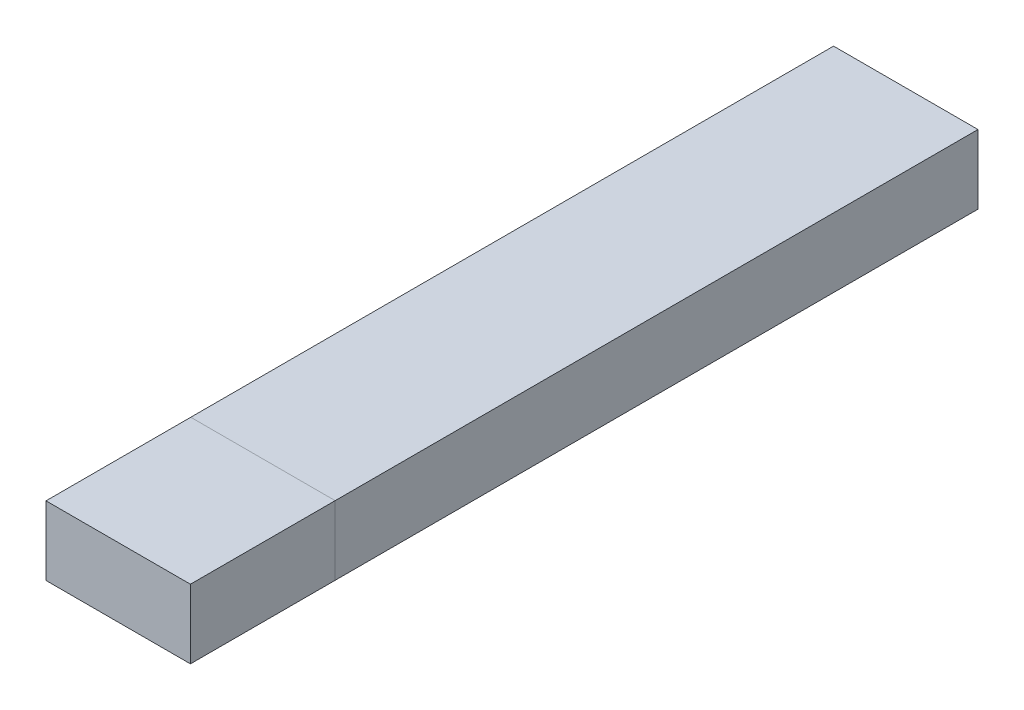
# Autodesk Inventor part: Contenedor3
Saved by Autodesk Inventor 2020.3 (Build 243373000, 373)
## iProperties
Created: 2020-09-22
Part Number: Contenedor3
Material: ABS Plastic
Document SubType Name: Modeling
Designer: juanp
Density: 1.06 g/cm^3
Appearance: Smooth - White
Mass: 443.385 g
Surface Area: 3011.82 cm^2
Volume: 418.287 cm^3
Author: juanp
Autodesk Inventor part; units mm, degrees
sketch "Sketch1" plane through (0, 0, 0) normal (0, 1, 0) x (-1, 0, 0)
  line L0 (0, 0) -> (0, -358.09) construction
  line L1 (42, 13.6996) -> (0, 13.6996)
  line L2 (0, 13.6996) -> (0, -13.6996)
  line L3 (0, -13.6996) -> (42, -13.6996)
  line L4 (42, -13.6996) -> (42, 13.6996)
  line L5 (42, -15.6996) -> (0, -15.6996)
  line L6 (0, -15.6996) -> (0, -43.0987)
  line L7 (0, -43.0987) -> (42, -43.0987)
  line L8 (42, -43.0987) -> (42, -15.6996)
  line L9 (42, -45.0987) -> (0, -45.0987)
  line L10 (0, -45.0987) -> (0, -72.4978)
  line L11 (0, -72.4978) -> (42, -72.4978)
  line L12 (42, -72.4978) -> (42, -45.0987)
  line L13 (42, -105.897) -> (0, -105.897)
  line L14 (0, -105.897) -> (0, -133.2961)
  line L15 (0, -133.2961) -> (42, -133.2961)
  line L16 (42, -133.2961) -> (42, -105.897)
  line L17 (42, -135.2961) -> (0, -135.2961)
  line L18 (0, -135.2961) -> (0, -162.6952)
  line L19 (0, -162.6952) -> (42, -162.6952)
  line L20 (42, -162.6952) -> (42, -135.2961)
  line L21 (42, -76.4978) -> (0, -76.4978)
  line L22 (0, -76.4978) -> (0, -103.897)
  line L23 (0, -103.897) -> (42, -103.897)
  line L24 (42, -103.897) -> (42, -76.4978)
  line L25 (21, -13.6996) -> (21, -15.6996)
  line L26 (21, -43.0987) -> (21, -45.0987)
  line L27 (21, -103.897) -> (21, -105.897)
  line L28 (21, -133.2961) -> (21, -135.2961)
  line L29 (42, -166.6952) -> (0, -166.6952)
  line L30 (0, -166.6952) -> (0, -194.0943)
  line L31 (0, -194.0943) -> (42, -194.0943)
  line L32 (42, -194.0943) -> (42, -166.6952)
  line L33 (42, -196.0943) -> (0, -196.0943)
  line L34 (0, -196.0943) -> (0, -223.4935)
  line L35 (0, -223.4935) -> (42, -223.4935)
  line L36 (42, -223.4935) -> (42, -196.0943)
  line L37 (42, -225.4935) -> (0, -225.4935)
  line L38 (0, -225.4935) -> (0, -252.8926)
  line L39 (0, -252.8926) -> (42, -252.8926)
  line L40 (42, -252.8926) -> (42, -225.4935)
  line L41 (42, -286.2917) -> (0, -286.2917)
  line L42 (0, -286.2917) -> (0, -313.6909)
  line L43 (0, -313.6909) -> (42, -313.6909)
  line L44 (42, -313.6909) -> (42, -286.2917)
  line L45 (42, -315.6909) -> (0, -315.6909)
  line L46 (0, -315.6909) -> (0, -343.09)
  line L47 (0, -343.09) -> (42, -343.09)
  line L48 (42, -343.09) -> (42, -315.6909)
  line L49 (42, -256.8926) -> (0, -256.8926)
  line L50 (0, -256.8926) -> (0, -284.2917)
  line L51 (0, -284.2917) -> (42, -284.2917)
  line L52 (42, -284.2917) -> (42, -256.8926)
  line L53 (21, -194.0943) -> (21, -196.0943)
  line L54 (21, -223.4935) -> (21, -225.4935)
  line L55 (21, -284.2917) -> (21, -286.2917)
  line L56 (21, -313.6909) -> (21, -315.6909)
  line L57 (88, 15.6996) -> (-2, 15.6996)
  line L58 (-2, 15.6996) -> (-2, -475.09)
  line L59 (-2, -475.09) -> (88, -475.09)
  line L60 (88, -475.09) -> (88, 15.6996)
  line L61 (44, 0) -> (44, -362.09) construction
  line L62 (86, 13.6996) -> (44, 13.6996)
  line L63 (44, 13.6996) -> (44, -13.6996)
  line L64 (44, -13.6996) -> (86, -13.6996)
  line L65 (86, -13.6996) -> (86, 13.6996)
  line L66 (86, -15.6996) -> (44, -15.6996)
  line L67 (44, -15.6996) -> (44, -43.0987)
  line L68 (44, -43.0987) -> (86, -43.0987)
  line L69 (86, -43.0987) -> (86, -15.6996)
  line L70 (86, -45.0987) -> (44, -45.0987)
  line L71 (44, -45.0987) -> (44, -72.4978)
  line L72 (44, -72.4978) -> (86, -72.4978)
  line L73 (86, -72.4978) -> (86, -45.0987)
  line L74 (86, -105.897) -> (44, -105.897)
  line L75 (44, -105.897) -> (44, -133.2961)
  line L76 (44, -133.2961) -> (86, -133.2961)
  line L77 (86, -133.2961) -> (86, -105.897)
  line L78 (86, -135.2961) -> (44, -135.2961)
  line L79 (44, -135.2961) -> (44, -162.6952)
  line L80 (44, -162.6952) -> (86, -162.6952)
  line L81 (86, -162.6952) -> (86, -135.2961)
  line L82 (86, -76.4978) -> (44, -76.4978)
  line L83 (44, -76.4978) -> (44, -103.897)
  line L84 (44, -103.897) -> (86, -103.897)
  line L85 (86, -103.897) -> (86, -76.4978)
  line L86 (65, -13.6996) -> (65, -15.6996)
  line L87 (65, -43.0987) -> (65, -45.0987)
  line L88 (65, -103.897) -> (65, -105.897)
  line L89 (65, -133.2961) -> (65, -135.2961)
  line L90 (44, -225.4935) -> (44, -252.8926)
  line L91 (86, -252.8926) -> (86, -225.4935)
  line L92 (86, -256.8926) -> (44, -256.8926)
  line L93 (44, -256.8926) -> (44, -284.2917)
  line L94 (86, -284.2917) -> (86, -256.8926)
  line L95 (44, -252.8926) -> (86, -252.8926)
  line L96 (86, -166.6952) -> (44, -166.6952)
  line L97 (44, -166.6952) -> (44, -194.0943)
  line L98 (44, -194.0943) -> (86, -194.0943)
  line L99 (86, -194.0943) -> (86, -166.6952)
  line L100 (86, -225.4935) -> (44, -225.4935)
  line L101 (65, -223.4935) -> (65, -225.4935)
  line L102 (44, -223.4935) -> (86, -223.4935)
  line L103 (86, -223.4935) -> (86, -196.0943)
  line L104 (86, -196.0943) -> (44, -196.0943)
  line L105 (44, -196.0943) -> (44, -223.4935)
  line L106 (65, -194.0943) -> (65, -196.0943)
  line L107 (86, -286.2917) -> (44, -286.2917)
  line L108 (44, -286.2917) -> (44, -313.6909)
  line L109 (44, -313.6909) -> (86, -313.6909)
  line L110 (86, -313.6909) -> (86, -286.2917)
  line L111 (44, -284.2917) -> (86, -284.2917)
  line L112 (65, -313.6909) -> (65, -315.6909)
  line L113 (86, -315.6909) -> (44, -315.6909)
  line L114 (86, -343.09) -> (86, -315.6909)
  line L115 (44, -343.09) -> (86, -343.09)
  line L116 (44, -315.6909) -> (44, -343.09)
  line L117 (65, -284.2917) -> (65, -286.2917)
  line L118 (65, 13.6996) -> (65, 15.6996)
  line L119 (65, -72.4978) -> (65, -76.4978)
  line L120 (21, -72.4978) -> (21, -76.4978)
  line L121 (65, -162.6952) -> (65, -166.6952)
  line L122 (21, -162.6952) -> (21, -166.6952)
  line L123 (65, -252.8926) -> (65, -256.8926)
  line L124 (21, -252.8926) -> (21, -256.8926)
  line L125 (0, -347.09) -> (86, -347.09)
  line L126 (86, -347.09) -> (86, -377.09)
  line L127 (86, -377.09) -> (0, -377.09)
  line L128 (0, -377.09) -> (0, -347.09)
  line L129 (86, -362.09) -> (0, -362.09) construction
  line L130 (65, -343.09) -> (65, -347.09)
  line L131 (21, -343.09) -> (21, -347.09)
  line L132 (0, -379.09) -> (86, -379.09)
  line L133 (86, -379.09) -> (86, -409.09)
  line L134 (86, -409.09) -> (0, -409.09)
  line L135 (0, -409.09) -> (0, -379.09)
  line L136 (0, -411.09) -> (86, -411.09)
  line L137 (86, -411.09) -> (86, -441.09)
  line L138 (86, -441.09) -> (0, -441.09)
  line L139 (0, -441.09) -> (0, -411.09)
  line L140 (43, -377.09) -> (43, -379.09)
  line L141 (43, -409.09) -> (43, -411.09)
  line L142 (0, -443.09) -> (86, -443.09)
  line L143 (86, -443.09) -> (86, -473.09)
  line L144 (86, -473.09) -> (0, -473.09)
  line L145 (0, -473.09) -> (0, -443.09)
  line L146 (43, -441.09) -> (43, -443.09)
  line L147 (43, -475.09) -> (43, -473.09)
  point P0 (0, -29.3991)
  point P1 (0, -58.7983)
  point P2 (0, -119.5965)
  point P3 (0, -148.9957)
  point P4 (0, -90.1974)
  point P5 (0, -180.3948)
  point P6 (0, -209.7939)
  point P7 (0, -239.193)
  point P8 (0, -299.9913)
  point P9 (0, -329.3904)
  point P10 (0, -270.5922)
  point P11 (44, -29.3991)
  point P12 (44, -58.7983)
  point P13 (44, -119.5965)
  point P14 (44, -148.9957)
  point P15 (44, -90.1974)
  point P16 (44, -239.193)
  point P17 (44, -270.5922)
  point P18 (44, -180.3948)
  point P19 (44, -209.7939)
  point P20 (44, -299.9913)
  point P21 (44, -329.3904)
  point P22 (65, -254.8926)
  point P23 (0, -458.09)
  dimension "d7" = 2
  dimension "d8" = 2
  dimension "d12" = 2
  dimension "d13" = 2
  dimension "d14" = 90
  dimension "d15" = 2
  dimension "d16" = 4
  dimension "d17" = 4
  dimension "d18" = 4
  dimension "d25" = 30
  dimension "d27" = 27.3991
  dimension "d28" = 92.1974
  dimension "d30" = 458.09
  constraints: 292 end point, 83 midpoint, 73 equal length, 58 parallel, 32 perpendicular, 29 horizontal, 6 point on line, 5 collinear, 1 coincident, 29 other
  measures "d7" distance between parallel lines of L58 L2
  measures "d8" distance between parallel lines of L57 L1
  measures "d12" distance of L118.start L118.end
  measures "d13" distance between parallel lines of L60 L73
  measures "d14" distance of L58.end L59.end
  measures "d15" distance between parallel lines of L4 L63
  measures "d16" distance of L120.start L120.end
  measures "d17" distance of L122.start L122.end
  measures "d18" distance of L124.start L124.end
  measures "d25" distance of L125.end L126.end
  measures "d27" distance of L48.start L45.start
  measures "d28" distance from line of point (65, -254.893) L125
  measures "d30" distance of point (0, 0) point (0, -458.09)
extrude "Extrusion1" add sketch "Sketch1" along normal blind 40 contours L60 L59 L147 L144 L143 L142 L146 L138 L137 L136 L141 L134 L133 L132 L140 L127 L126 L125 L130 L115 L114 L113 L112 L109 L110 L107 L117 L111 L94 L92 L123 L95 L91 L100 L101 L102 L103 L104 L106 L98 L99 L96 L121 L80 L81 L78 L89 L76 L77 L74 L88 L84 L85 L82 L119 L72 L73 L70 L87 L68 L69 L66 L86 L64 L65 L62 L118 L57 | L118 L62 L63 L64 L86 L66 L67 L68 L87 L70 L71 L72 L119 L82 L83 L84 L88 L74 L75 L76 L89 L78 L79 L80 L121 L96 L97 L98 L106 L104 L105 L102 L101 L100 L90 L95 L123 L92 L93 L111 L117 L107 L108 L109 L112 L113 L116 L115 L130 L125 L128 L127 L140 L132 L135 L134 L141 L136 L139 L138 L146 L142 L145 L144 L147 L59 L58 L57
sketch "Sketch2" plane through (0, 40, 0) normal (0, 1, 0) x (1, 0, 0)
  line L0 (2, -15.6996) -> (2, 475.09) projected
  line L1 (-88, -15.6996) -> (2, -15.6996) projected
  line L2 (-88, 475.09) -> (-88, -15.6996) projected
  line L3 (2, 475.09) -> (-88, 475.09) projected
  point P0 (0, 0)
extrude "Extrusion2" add sketch "Sketch2" along normal blind 3
fillet "Fillet1" radius 5 192 edges at (-42, 20, -45.0987) (0, 20, -45.0987) (-42, 20, -43.0987) (0, 20, -15.6996) (-21, 40, 13.6996) (-44, 20, -103.897) (-44, 20, -105.897) (-44, 20, -133.2961) (-86, 20, -133.2961) (-86, 20, -105.897) (-86, 20, -76.4978) (0, 20, -72.4978) (-21, 40, -43.0987) (-86, 20, -13.6996) (-86, 20, -15.6996) (-44, 20, -15.6996) (-86, 20, 13.6996) (-44, 20, -13.6996) (-44, 20, 13.6996) (-42, 20, -15.6996) (-86, 40, -270.5922) (-42, 40, -299.9913) (-65, 40, -286.2917) (-86, 40, -299.9913) (-44, 40, -299.9913) (-42, 40, -270.5922) (-44, 40, -270.5922) (-42, 40, -239.193) (-65, 40, -284.2917) (-65, 40, -313.6909) (0, 20, -43.0987) (-42, 40, -29.3991) (-21, 40, -15.6996) (-42, 20, -13.6996) (0, 20, -13.6996) (0, 20, 13.6996) (0, 20, -162.6952) (0, 20, -135.2961) (0, 20, -133.2961) (-42, 20, -162.6952) (-42, 20, -135.2961) (-86, 20, -135.2961) (-44, 20, -135.2961) (-86, 20, -162.6952) (-44, 20, -162.6952) (-86, 20, -166.6952) (-44, 40, -180.3948) (0, 20, -194.0943) (-42, 20, -166.6952) (-42, 20, -194.0943) (0, 20, -166.6952) (-44, 20, -43.0987) (-44, 20, -45.0987) (-44, 20, -72.4978) (-44, 20, -76.4978) (-86, 20, -43.0987) (-86, 20, -45.0987) (-21, 40, -13.6996) (-86, 20, -72.4978) (-42, 20, 13.6996) (-86, 20, -103.897) (-65, 40, -223.4935) (-86, 40, -209.7939) (-65, 40, -196.0943) (-44, 40, -209.7939) (-65, 40, -166.6952) (-65, 40, -194.0943) (-86, 40, -180.3948) (-65, 40, -162.6952) (-44, 20, -166.6952) (-86, 20, -194.0943) (-86, 20, -196.0943) (-86, 20, -223.4935) (-44, 20, -223.4935) (-44, 20, -194.0943) (0, 20, -223.4935) (0, 20, -196.0943) (-42, 20, -196.0943) (-42, 20, -223.4935) (-42, 40, -180.3948) (0, 40, -180.3948) (-21, 40, -196.0943) (-21, 40, -223.4935) (-42, 40, -209.7939) (0, 40, -209.7939) (-21, 40, -225.4935) (0, 40, -239.193) (-21, 40, -194.0943) (-44, 20, -196.0943) (-86, 20, -225.4935) (-44, 20, -225.4935) (-86, 20, -252.8926) (-44, 20, -252.8926) (-86, 20, -256.8926) (-65, 40, -256.8926) (-65, 40, -252.8926) (-86, 40, -239.193) (-44, 40, -239.193) (-65, 40, -225.4935) (0, 20, -252.8926) (0, 20, -225.4935) (-42, 20, -252.8926) (-42, 20, -225.4935) (-86, 20, -284.2917) (0, 20, -313.6909) (0, 20, -286.2917) (-42, 20, -286.2917) (-42, 20, -313.6909) (-44, 20, -256.8926) (-44, 20, -284.2917) (-44, 20, -286.2917) (-44, 20, -313.6909) (-86, 20, -313.6909) (-86, 20, -286.2917) (-42, 20, -315.6909) (-42, 20, -343.09) (0, 20, -315.6909) (-44, 20, -315.6909) (-86, 20, -315.6909) (-44, 20, -343.09) (-86, 20, -343.09) (0, 20, -343.09) (-21, 40, -252.8926) (-21, 40, -256.8926) (0, 40, -270.5922) (-21, 40, -284.2917) (0, 40, -299.9913) (-21, 40, -286.2917) (-21, 40, -313.6909) (-21, 40, -315.6909) (-65, 40, -315.6909) (-42, 40, -329.3904) (-21, 40, -343.09) (0, 40, -329.3904) (-44, 40, -329.3904) (-86, 40, -329.3904) (-65, 40, -343.09) (0, 20, -284.2917) (0, 20, -256.8926) (-42, 20, -256.8926) (-42, 20, -284.2917) (-65, 40, -72.4978) (-86, 40, -58.7983) (-65, 40, -45.0987) (-44, 40, -58.7983) (-65, 40, -43.0987) (-86, 40, -29.3991) (-65, 40, -15.6996) (-44, 40, -29.3991) (-65, 40, -13.6996) (-86, 40, 0) (-65, 40, 13.6996) (-44, 40, 0) (-44, 40, -148.9957) (-86, 40, -148.9957) (-65, 40, -133.2961) (-65, 40, -135.2961) (-86, 40, -119.5965) (-44, 40, -119.5965) (-65, 40, -105.897) (-21, 40, -133.2961) (-21, 40, -135.2961) (0, 40, -148.9957) (-21, 40, -162.6952) (-42, 40, -148.9957) (-21, 40, -105.897) (0, 40, -119.5965) (-42, 40, -119.5965) (-21, 40, -103.897) (-21, 40, -76.4978) (-42, 40, -90.1974) (0, 40, -90.1974) (-21, 40, -166.6952) (-42, 20, -72.4978) (-42, 20, -133.2961) (0, 20, -105.897) (-42, 20, -105.897) (0, 20, -103.897) (-42, 20, -103.897) (-21, 40, -45.0987) (0, 40, -58.7983) (-42, 40, -58.7983) (-21, 40, -72.4978) (0, 40, -29.3991) (-42, 40, 0) (0, 40, 0) (0, 20, -76.4978) (-42, 20, -76.4978) (-86, 40, -90.1974) (-65, 40, -76.4978) (-44, 40, -90.1974) (-65, 40, -103.897)
ref_plane "Work Plane1" through (-88, 0, -229.6952) normal (0, 0, 1) x (1, 0, 0)
ref_plane "Work Plane2" through (-43, 0, 15.6996) normal (1, 0, 0) x (0, 0, -1)
ref_plane "Work Plane3" through (-43, 0, 15.6996) normal (1, 0, 0) x (0, 0, -1)
ref_plane "Work Plane4" through (-81, 0, -74.4978) normal (0, 0, 1) x (1, 0, 0)
ref_plane "Work Plane5" through (-49, 0, -164.6952) normal (0, 0, -1) x (-1, 0, 0)
ref_plane "Work Plane6" through (-49, 0, -254.8926) normal (0, 0, -1) x (-1, 0, 0)
ref_plane "Work Plane7" through (-81, 0, -345.09) normal (0, 0, 1) x (1, 0, 0)
ref_plane "Work Plane8" through (-81, 0, -29.3991) normal (0, 0, 1) x (1, 0, 0)
ref_plane "Work Plane9" through (-81, 0, -18.3991) normal (0, 0, 1) x (1, 0, 0)
sketch "Sketch8" plane through (-81, 0, -18.3991) normal (0, 0, 1) x (1, 0, 0)
  line L0 (-7, 2) -> (-7, 43)
  line L1 (-7, 2) -> (-19.5, 2)
  line L2 (-19.5, 2) -> (-19.5, 34.1)
  line L3 (-19.5, 34.1) -> (-7, 34.1)
  line L4 (-7, 34.1) -> (-7, 2)
  line L5 (-7, 29.5) -> (-19.5, 29.5)
  line L6 (-7, 6.6) -> (-19.5, 6.6)
  line L7 (-19.5, 34.1) -> (-22.5, 34.1)
  line L8 (-22.5, 34.1) -> (-22.5, 2)
  line L9 (-22.5, 2) -> (-19.5, 2)
  line L10 (-19.5, 2) -> (-19.5, 34.1)
  line L11 (-7, 43) -> (-22.5, 34.1)
  line L12 (-7, 0) -> (-7, 2)
  line L13 (-7, 0) -> (-7, 43)
  line L14 (83, 43) -> (-7, 43) projected
  point P0 (81, 0)
  point P1 (-7, 34.1)
  point P2 (-19.5, 2)
  dimension "d59" = 12.5
  dimension "d60" = 32.1
  dimension "d61" = 4.6
  dimension "d62" = 4.6
  dimension "d63" = 3
  dimension "d64" = 2
  constraints: 28 end point, 5 point on line, 4 parallel, 4 perpendicular, 2 horizontal, 1 coincident, 1 collinear, 1 vertical
  measures "d59" distance of L2.end L3.end
  measures "d60" distance of L1.end L2.end
  measures "d61" distance between parallel lines of L5 L3
  measures "d62" distance between parallel lines of L1 L6
  measures "d63" distance between parallel lines of L8 L2
  measures "d64" distance of L12.start L1.start
extrude "Extrusion7" [suppressed]
pattern_linear "Rectangular Pattern2" [suppressed]
split body "Split6" result two bodies by plane through (-81, 0, -74.4978) normal (0, 0, 1) first body at (-58, 42.5, -44.432)
body "Solid12"
body "Solid13"
